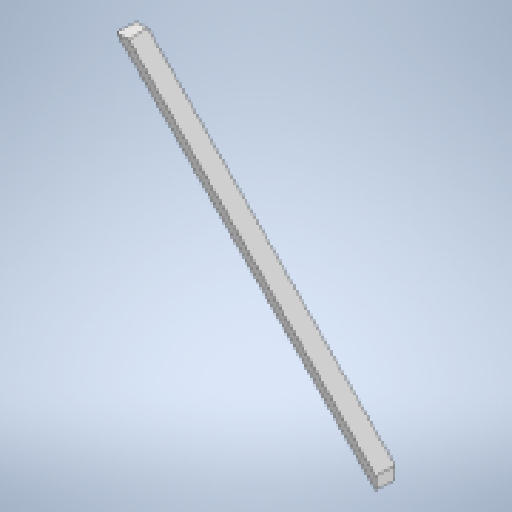
# Autodesk Inventor part: side-side
Saved by Autodesk Inventor 2025.1 (Build 291241020, 241B)
## iProperties
Created: 2024-09-20
Part Number: side-side
Material: Generic
Document SubType Name: Modeling
Designer: User
Density: 1 g/cm^3
Appearance: Default
Author: User
Autodesk Inventor part; units mm, degrees
ref_plane "YZ Plane" through (0, 0, 0) normal (1, 0, 0) x (0, 1, 0)
ref_plane "XZ Plane" through (0, 0, 0) normal (0, 1, 0) x (-1, 0, 0)
ref_plane "XY Plane" through (0, 0, 0) normal (0, 0, 1) x (1, 0, 0)
sketch "Sketch1" plane through (0, 0, 0) normal (0, 0, 1) x (1, 0, 0)
  line L0 (0, 0) -> (0, 1219.2) projected
  line L1 (-1181.1, 1219.2) -> (38.1, 1219.2) projected
  line L2 (-1181.1, 1219.2) -> (0, 0)
  line L3 (0, 54.7575) -> (-1128.0537, 1219.2)
  line L4 (-1181.1, 1219.2) -> (-1128.0537, 1219.2)
  line L5 (-1128.0537, 1219.2) -> (-1181.1, 1219.2)
  dimension "d0" = 38.1
  constraints: 8 end point, 2 collinear, 2 point on line, 1 parallel
  measures "d0" distance between parallel lines of L2 L3
extrude "Extrusion1" add sketch "Sketch1" against normal blind 88.9 contours L2 L1 L3 L0
body "Solid1"
